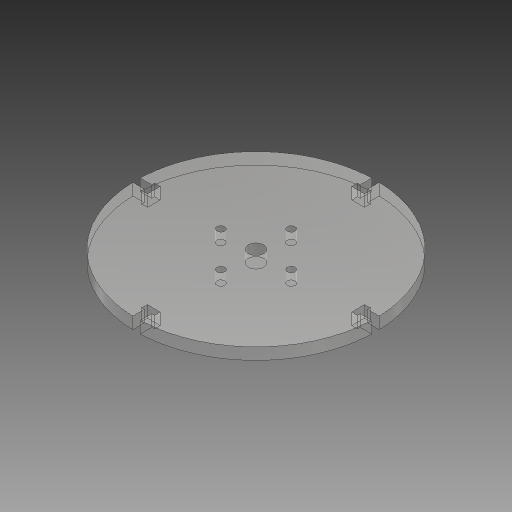
# Autodesk Inventor part: PlexiHalter2
Saved by Autodesk Inventor 2019 (Build 230136000, 136)
## iProperties
Created: 2018-05-15
Part Number: PlexiHalter2
Material: Polycarbonate, Clear
Document SubType Name: Modeling
Designer: Phil Erle
Density: 1.2 g/cm^3
Appearance: Polycarbonate - Clear
Author: Phil Erle
Autodesk Inventor part; units mm, degrees
ref_plane "YZ Plane" through (0, 0, 0) normal (1, 0, 0) x (0, 1, 0)
ref_plane "XZ Plane" through (0, 0, 0) normal (0, 1, 0) x (-1, 0, 0)
ref_plane "XY Plane" through (0, 0, 0) normal (0, 0, 1) x (1, 0, 0)
sketch "Sketch1" plane through (0, 0, 0) normal (0, 0, 1) x (1, 0, 0)
  circle A0 centre (0, 0) radius 51
  dimension "d0" = 102
  constraints: 1 centre point, 1 coincident
  measures "d0" diameter of A0
extrude "Extrusion1" add sketch "Sketch1" along normal blind 5
sketch "Sketch2" plane through (0, 0, 5) normal (0, 0, 1) x (1, 0, 0)
  point P0 (0, 0)
  point P1 (0, 0)
  constraints: 1 coincident
hole "Hole1" at (0, 0, 5) direction (0, 0, -1) diameter 6.6 depth 8 tip angle 118 clearance for "Countersunk Flat Head Screw DIN EN ISO 2009" size "M6" standard "DIN"
sketch "Sketch3" plane through (0, 0, 5) normal (0, 0, 1) x (1, 0, 0)
  circle A0 centre (0, 0) radius 15 construction
  point P0 (-15, 0)
  point P1 (0, 15)
  point P2 (15, 0)
  point P3 (0, -15)
  dimension "d10" = 30
  constraints: 4 point on circle, 2 horizontal alignment, 2 vertical alignment, 1 centre point, 1 coincident
  measures "d10" diameter of A0
hole "Hole2" at (-15, 0, 5) at (0, 15, 5) at (15, 0, 5) at (0, -15, 5) direction (0, 0, -1) diameter 3.4 depth 8 tip angle 118 clearance for "Countersunk Flat Head Screw DIN EN ISO 2009" size "M3" standard "DIN"
sketch "Sketch4" plane through (0, 0, 5) normal (0, 0, 1) x (1, 0, 0)
  line L0 (-51, 1.6) -> (-51, -1.6)
  line L1 (-51, -1.6) -> (-46, -1.6)
  line L2 (-46, -1.6) -> (-46, -2.75)
  line L3 (-46, -2.75) -> (-43.6, -2.75)
  line L4 (-43.6, -2.75) -> (-43.6, 2.75)
  line L5 (-43.6, 2.75) -> (-46, 2.75)
  line L6 (-46, 2.75) -> (-46, 1.6)
  line L7 (-46, 1.6) -> (-51, 1.6)
  line L8 (-1.6, -51) -> (1.6, -51)
  line L9 (1.6, -51) -> (1.6, -46)
  line L10 (1.6, -46) -> (2.75, -46)
  line L11 (2.75, -46) -> (2.75, -43.6)
  line L12 (2.75, -43.6) -> (-2.75, -43.6)
  line L13 (-2.75, -43.6) -> (-2.75, -46)
  line L14 (-2.75, -46) -> (-1.6, -46)
  line L15 (-1.6, -46) -> (-1.6, -51)
  line L16 (51, -1.6) -> (51, 1.6)
  line L17 (51, 1.6) -> (46, 1.6)
  line L18 (46, 1.6) -> (46, 2.75)
  line L19 (46, 2.75) -> (43.6, 2.75)
  line L20 (43.6, 2.75) -> (43.6, -2.75)
  line L21 (43.6, -2.75) -> (46, -2.75)
  line L22 (46, -2.75) -> (46, -1.6)
  line L23 (46, -1.6) -> (51, -1.6)
  line L24 (1.6, 51) -> (-1.6, 51)
  line L25 (-1.6, 51) -> (-1.6, 46)
  line L26 (-1.6, 46) -> (-2.75, 46)
  line L27 (-2.75, 46) -> (-2.75, 43.6)
  line L28 (-2.75, 43.6) -> (2.75, 43.6)
  line L29 (2.75, 43.6) -> (2.75, 46)
  line L30 (2.75, 46) -> (1.6, 46)
  line L31 (1.6, 46) -> (1.6, 51)
  point P0 (0, 0)
  point P1 (-43.6, 0)
  point P2 (-51, 0)
  point P3 (0, -51)
  point P4 (0, -43.6)
  point P5 (51, 0)
  point P6 (43.6, 0)
  point P7 (0, 51)
  point P8 (0, 43.6)
  dimension "d18" = 5.5
  dimension "d19" = 5
  dimension "d20" = 2.4
  dimension "d21" = 3.2
  dimension "d22" = 51
  dimension "d25" = 360
  constraints: 64 end point, 8 point on line, 4 perpendicular, 3 horizontal alignment, 2 midpoint, 1 parallel, 1 vertical, 73 other
  measures "d18" distance of L3.end L4.end
  measures "d19" distance of L6.end L0.start
  measures "d20" distance of L4.end L5.end
  measures "d21" distance of L0.start L0.end
  measures "d22" distance of point (0, 0) point (-51, 0)
extrude "Extrusion2" cut sketch "Sketch4" against normal through all
equation "\"d27\" = d22"
body "Solid1"
